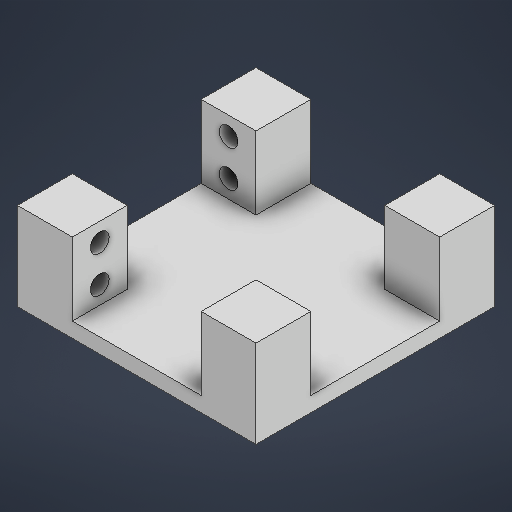
# Autodesk Inventor part: Ruler square
Saved by Autodesk Inventor 2027 (Build 310192060, 192F)
## iProperties
Created: 2026-06-30
Part Number: Ruler square
Material: Generic
Document SubType Name: Modeling
Designer: blaze
Density: 1 g/cm^3
Appearance: Default
Author: blaze
Autodesk Inventor part; units mm, degrees
ref_plane "YZ Plane" through (0, 0, 0) normal (1, 0, 0) x (0, 1, 0)
ref_plane "XZ Plane" through (0, 0, 0) normal (0, 1, 0) x (-1, 0, 0)
ref_plane "XY Plane" through (0, 0, 0) normal (0, 0, 1) x (1, 0, 0)
sketch "Sketch1" plane through (0, 0, 0) normal (0, 0, 1) x (1, 0, 0)
  line L0 (0, 0) -> (50.8, 0)
  line L1 (50.8, 0) -> (50.8, 3.175)
  line L2 (50.8, 3.175) -> (0, 3.175)
  line L3 (0, 3.175) -> (0, 0)
  line L4 (0, 3.175) -> (11.684, 3.175)
  line L5 (11.684, 3.175) -> (11.684, 18.669)
  line L6 (11.684, 18.669) -> (0, 18.669)
  line L7 (0, 18.669) -> (0, 3.175)
  line L8 (50.8, 3.175) -> (39.116, 3.175)
  line L9 (39.116, 3.175) -> (39.116, 18.669)
  line L10 (39.116, 18.669) -> (50.8, 18.669)
  line L11 (50.8, 18.669) -> (50.8, 3.175)
  dimension "d0" = 50.8
  dimension "d1" = 3.175
  dimension "d2" = 11.684
  dimension "d3" = 15.494
  dimension "d4" = 11.684
  dimension "d5" = 15.494
  constraints: 24 end point, 6 parallel, 3 horizontal, 3 perpendicular
  measures "d0" distance of L2.end L1.end
  measures "d1" distance of L1.end L0.end
  measures "d2" distance of L6.end L5.end
  measures "d3" distance of L5.end L4.end
  measures "d4" distance of L9.end L10.end
  measures "d5" distance of L8.end L9.end
extrude "Extrusion1" add sketch "Sketch1" against normal blind 50.8
sketch "Sketch2" plane through (50.8, 0, 0) normal (1, 0, 0) x (0, 0, -1)
  line L0 (0, 3.175) -> (0, 18.669) projected
  line L1 (0, 3.175) -> (11.684, 3.175)
  line L2 (11.684, 3.175) -> (11.684, 18.669)
  line L3 (11.684, 18.669) -> (0, 18.669)
  line L4 (0, 18.669) -> (0, 3.175)
  line L5 (0, 18.669) -> (50.8, 18.669) projected
  line L6 (0, 3.175) -> (50.8, 3.175) projected
  line L7 (50.8, 18.669) -> (39.116, 18.669)
  line L8 (39.116, 18.669) -> (39.116, 3.175)
  line L9 (39.116, 3.175) -> (50.8, 3.175)
  line L10 (50.8, 3.175) -> (50.8, 18.669)
  line L11 (11.684, 3.175) -> (39.116, 3.175)
  point P0 (0, 0)
  dimension "d8" = 11.684
  dimension "d9" = 15.494
  dimension "d10" = 11.684
  constraints: 18 end point, 4 parallel, 2 horizontal, 2 perpendicular, 1 collinear, 1 point on line
  measures "d8" distance of L3.end L2.end
  measures "d9" distance of L2.end L1.end
  measures "d10" distance of L9.end L8.end
extrude "Extrusion2" cut sketch "Sketch2" against normal blind 50.8 contours L2 L5 L8 L6
sketch "Sketch3" plane through (0, 0, 0) normal (-1, 0, 0) x (0, 0, 1)
  line L0 (0, 3.175) -> (-11.684, 3.175) projected
  circle A0 centre (-5.842, 6.985) radius 2
  line L1 (0, 3.175) -> (0, 18.669) projected
  circle A1 centre (-5.842, 14.732) radius 2
  point P0 (0, 0)
  dimension "d14" = 4
  dimension "d16" = 4
  constraints: 2 centre point
  measures "d14" diameter of A0
  measures "d16" diameter of A1
extrude "Extrusion3" cut sketch "Sketch3" against normal up to surface (11.684 mm away)
sketch "Sketch4" plane through (0, 0, -50.8) normal (0, 0, -1) x (-1, 0, 0)
  line L0 (-11.684, 3.175) -> (0, 3.175) projected
  circle A0 centre (-5.842, 6.985) radius 2
  line L1 (-11.684, 3.175) -> (-11.684, 18.669) projected
  line L2 (0, 18.669) -> (0, 3.175) projected
  circle A1 centre (-5.842, 14.732) radius 2
  point P0 (0, 0)
  dimension "d20" = 4
  dimension "d22" = 4
  constraints: 2 centre point
  measures "d20" diameter of A0
  measures "d22" diameter of A1
extrude "Extrusion4" cut sketch "Sketch4" against normal up to surface (11.684 mm away)
body "Solid1"
